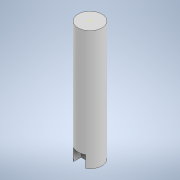
# Autodesk Inventor part: ADJ_shaft_v2
Saved by Autodesk Inventor 2021 (Build 250183000, 183)
## iProperties
Created: 2021-10-31
Part Number: ADJ_shaft_v2
Material: Generic
Document SubType Name: Modeling
Designer: shubh
Density: 1 g/cm^3
Appearance: Default
Author: shubh
Autodesk Inventor part; units mm, degrees
sketch "Sketch1" plane through (0, 0, 0) normal (0, 1, 0) x (-1, 0, 0)
  circle A0 centre (0, 0) radius 2.54
  dimension "shaft_diameter" = 5.08
  constraints: 1 centre point, 1 coincident
  measures "shaft_diameter" diameter of A0
extrude "Extrusion1" add sketch "Sketch1" along normal blind 25.4
sketch "Sketch2" plane through (0, 25.4, 0) normal (0, 1, 0) x (1, 0, 0)
  point P0 (0, 0)
ref_plane "Work Plane1" through (0, 19.05, 0) normal (0, 1, 0) x (1, 0, 0)
ref_plane "Work Plane2" through (0, 6.35, 0) normal (0, 1, 0) x (1, 0, 0)
sketch "Sketch6" plane through (0, 0, 0) normal (0, 0, 1) x (1, 0, 0)
  point P0 (0, 0)
ref_plane "Work Plane3" through (0, 0, 10.16) normal (0, 0, 1) x (1, 0, 0)
sketch "Sketch8" plane through (0, 0, 0) normal (0, -1, 0) x (1, 0, 0)
  circle A0 centre (0, 0) radius 2.54 projected
  line L0 (-1.27, 2.1997) -> (-1.27, 0.635)
  line L1 (-1.27, 0.635) -> (1.27, 0.635)
  line L2 (1.27, 0.635) -> (1.27, 2.1997)
  dimension "d25" = 0.635
  dimension "d26" = 1.27
  constraints: 6 end point, 2 perpendicular, 2 point on circle, 1 parallel, 1 vertical
  measures "d25" distance from line of point (0, 0) L1
  measures "d26" distance from line of point (0, 0) L0
extrude "Extrusion6" cut sketch "Sketch8" against normal blind 2.54 contours L2 L1 L0 A0 picked at (0.0885, 1.2654)
body "Solid1"
